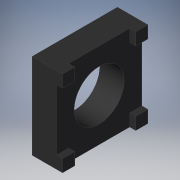
# Autodesk Inventor part: Robotunits GUS_4502
Saved by Autodesk Inventor 2019 (Build 230136000, 136)
## iProperties
Created: 2023-08-22
Part Number: Robotunits GUS_4502
Material: Generic
Catalog Web Link: www.cadenas.de
Description: GUS 4502-Angle
Vendor: ROBOTUNITS
Document SubType Name: Modeling
Designer: psAdmin
Manufacturer: ROBOTUNITS
Mass: 0.588759 g
Surface Area: 6.45424 cm^2
Volume: 0.588759 cm^3
Density: 1 g/cm^3
Appearance: PSOLRGB-175-175-175
Category: PARTsolutions
Company: ROBOTUNITS
Title: Robotunits GUS_4502
Author: Cadenas PARTsolutions
Comments: Angle
PSOL_IDENT_0: {$CADENAS_DATA/23d-libs/robotunits/profil_und_verbindungstechnik/verbindungstechnik_raster_40/parts/
PSOL_IDENT_1: gus_4502.prj},171 {VTYP=3D},{NB=Robotunits GUS_4502},{LINA=Robotunits GUS_4502},{NN=GUS 4502},{DATE=
PSOL_IDENT_2: 01.02.2021 08:30:03},{GEOMDATE=14.06.2007},{VERSION=},{LINEID=50},{WBVAR=},{WBNUMERIC=}  {NB=Robotun
PSOL_IDENT_3: its GUS_4502},{LINA=Robotunits GUS_4502},{KT=DUMMY},{ARTIKEL=GUS_4502},{M=M8},{NDM=8.000},{KDM=6.647
PSOL_IDENT_4: }
NB: Robotunits GUS_4502
NN: GUS 4502
NT: Angle
NBSYN: Robotunits $ARTIKEL.
LINA: Robotunits GUS_4502
CATALOG: Robotunits
ARTIKEL: GUS_4502
M: M8
NDM: 8
KDM: 6.647
SUPPLIER: ROBOTUNITS
ARTICLENO: Robotunits GUS_4502
BOMINFO: Robotunits GUS_4502
CREATOR: CADENAS GmbH
Autodesk Inventor part; units mm, degrees
sketch "Skizze_1" plane through (0, 0, 0) normal (1, 0, 0) x (0, 1, 0)
  line L0 (-7, 7) -> (-7, -7)
  line L1 (-7, -7) -> (7, -7)
  line L2 (7, -7) -> (7, 7)
  line L3 (7, 7) -> (-7, 7)
  circle A0 centre (0, 0) radius 4.1
  constraints: 8 end point, 1 centre point
extrude "Extrusion1" add sketch "Skizze_1" along normal blind 5
sketch "Skizze_2" plane through (5, 0, 0) normal (1, 0, 0) x (0, 0, -1)
  line L0 (-7, 5) -> (-7, -5)
  line L1 (-7, -5) -> (-5, -5)
  line L2 (-5, -5) -> (-5, -7)
  line L3 (-5, -7) -> (5, -7)
  line L4 (5, -7) -> (5, -5)
  line L5 (5, -5) -> (7, -5)
  line L6 (7, -5) -> (7, 5)
  line L7 (7, 5) -> (5, 5)
  line L8 (5, 5) -> (5, 7)
  line L9 (5, 7) -> (-5, 7)
  line L10 (-5, 7) -> (-5, 5)
  line L11 (-5, 5) -> (-7, 5)
  constraints: 24 end point
extrude "Extrusion2" cut sketch "Skizze_2" against normal blind 1
ref_plane "GUS_4502_1_XY" through (0, 0, 0) normal (1, 0, 0) x (0, 0, -1)
ref_plane "GUS_4502_1_YZ" through (0, 0, 0) normal (0, 0, -1) x (0, 1, 0)
ref_plane "GUS_4502_1_ZX" through (0, 0, 0) normal (0, 1, 0) x (1, 0, 0)
body "Solid1"
